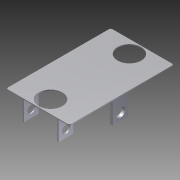
# Autodesk Inventor part: S114-electric
Saved by Autodesk Inventor 2011 SP1 (Build 150282100, 282)
## iProperties
Created: 2013-12-24
Part Number: S114-electric
Catalog Web Link: www.cadenas.de
Description: S Low Series electric-Low Capacity Standard Size Toggles -electric
Vendor: NKKSWITCHES
Document SubType Name: Modeling
Designer: PARTuser1
Manufacturer: NKKSWITCHES
Density: 1 g/cm^3
Category: PARTsolutions
Company: NKKSWITCHES
Title: S114-electric
Author: Cadenas PARTsolutions
Comments: Low Capacity Standard Size Toggles -electric
PSOL_IDENT_0: {$CADENAS_DATA\23d-libs\nkkswitches\toggle\s\parts\s_low_electric.prj},183 {VTYP=3D},{NB=S114-electr
PSOL_IDENT_1: ic},{LINA=S114-electric},{NN=S Low Series electric},{DATE=05.04.2013 12:38:11},{GEOMDATE=05.04.2013
PSOL_IDENT_2: 14:38:00},{VERSION=},{LINEID=10},{LINESUBID=-1},{WBVAR=}  {NB=S114-electric},{LINA=S114-electric},{K
PSOL_IDENT_3: T=DUMMY},{PN=S114},{MDL=S114}
CNS_NN: S Low Series electric
CNS_NT: Low Capacity Standard Size Toggles -electric
CNS_NB: S114-electric
CNS_NBSYN: $PN.-electric
CNS_LINA: S114-electric
CNS_PN: S114
CNS_MDL: S114
SUPPLIER: NKKSWITCHES
ARTICLENO: S114-electric
BOMINFO: S114-electric
CREATOR: CADENAS GmbH
Autodesk Inventor part; units mm, degrees
sketch "Sketch_1" plane through (0, 0, 0) normal (0, 1, 0) x (-1, 0, 0)
  line L0 (8.128, -12.954) -> (8.128, 12.954)
  arc A0 (8.128, 12.954) -> (7.62, 13.462) centre (7.62, 12.954) ccw
  line L1 (7.62, 13.462) -> (-7.62, 13.462)
  arc A1 (-7.62, 13.462) -> (-8.128, 12.954) centre (-7.62, 12.954) ccw
  line L2 (-8.128, 12.954) -> (-8.128, -12.954)
  arc A2 (-8.128, -12.954) -> (-7.62, -13.462) centre (-7.62, -12.954) ccw
  line L3 (-7.62, -13.462) -> (7.62, -13.462)
  arc A3 (7.62, -13.462) -> (8.128, -12.954) centre (7.62, -12.954) ccw
  circle A4 centre (0, 10.16) radius 3.048
  circle A5 centre (0, -10.16) radius 3.048
  constraints: 8 end point, 8 point on circle, 6 centre point
extrude "Extrusion1" add sketch "Sketch_1" along normal blind 0.254
sketch "Sketch_2" plane through (0, 0, 0) normal (0, 1, 0) x (1, 0, 0)
  line L0 (-4.6228, -12.7) -> (-4.318, -12.7)
  line L1 (-4.318, -12.7) -> (-4.318, -8.89)
  line L2 (-4.318, -8.89) -> (-4.6228, -8.89)
  line L3 (-4.6228, -8.89) -> (-4.6228, -12.7)
  constraints: 8 end point
extrude "Extrusion2" add sketch "Sketch_2" against normal blind 5.7658
sketch "Sketch_3" plane through (0, 0, 0) normal (0, 1, 0) x (1, 0, 0)
  line L0 (4.318, -12.7) -> (4.6228, -12.7)
  line L1 (4.6228, -12.7) -> (4.6228, -8.89)
  line L2 (4.6228, -8.89) -> (4.318, -8.89)
  line L3 (4.318, -8.89) -> (4.318, -12.7)
  constraints: 8 end point
extrude "Extrusion3" add sketch "Sketch_3" against normal blind 5.7658
sketch "Sketch4" plane through (-4.318, -5.7658, 8.89) normal (1, 0, 0) x (0, 0, -1)
  point P0 (-1.905, 1.9558)
hole "Drilling 1" at (-4.318, -3.81, 10.795) direction (-1, 0, 0) diameter 2.0066 depth 0.3048
sketch "Sketch5" plane through (4.318, -5.7658, 12.7) normal (-1, 0, 0) x (0, 0, 1)
  point P0 (-1.905, 1.9558)
hole "Drilling 2" at (4.318, -3.81, 10.795) direction (1, 0, 0) diameter 2.0066 depth 0.3048
sketch "Sketch_12" plane through (0, 0, 10.795) normal (0, 0, 1) x (1, 0, 0)
  line L0 (-4.6228, -1.27) -> (-4.9276, -1.27)
  arc A0 (-4.6228, -0.508) -> (-4.9276, -1.27) centre (-4.043, -1.1819) ccw
  line L1 (-4.6228, -0.508) -> (-4.6228, -1.27)
  line L2 (-4.6228, -1.27) -> (-4.9276, -1.27)
  constraints: 6 end point, 2 point on circle, 1 centre point
revolve "Revolution1" add sketch "Sketch_12" angle 360 about axis through (-4.6228, -1.27, 10.795) along (1, 0, 0)
sketch "Sketch_13" plane through (0, 0, 10.795) normal (0, 0, 1) x (1, 0, 0)
  line L0 (4.9276, -1.27) -> (4.6228, -1.27)
  line L1 (4.6228, -1.27) -> (4.6228, -0.508)
  arc A0 (4.9276, -1.27) -> (4.6228, -0.508) centre (4.043, -1.1819) ccw
  line L2 (4.9276, -1.27) -> (4.6228, -1.27)
  constraints: 6 end point, 2 point on circle, 1 centre point
revolve "Revolution2" add sketch "Sketch_13" angle 360 about axis through (4.9276, -1.27, 10.795) along (1, 0, 0)
sketch "Sketch_14" plane through (0, 0, 0) normal (0, 1, 0) x (-1, 0, 0)
  line L0 (7.8994, 1.9939) -> (7.112, 1.9939)
  line L1 (7.112, 1.9939) -> (7.112, -1.9939)
  line L2 (7.112, -1.9939) -> (7.8994, -1.9939)
  line L3 (7.8994, -1.9939) -> (7.8994, 1.9939)
  constraints: 8 end point
extrude "Extrusion4" add sketch "Sketch_14" against normal blind 5.7658
sketch "Sketch_15" plane through (0, 0, 0) normal (0, 1, 0) x (-1, 0, 0)
  line L0 (-7.112, 1.9939) -> (-7.8994, 1.9939)
  line L1 (-7.8994, 1.9939) -> (-7.8994, -1.9939)
  line L2 (-7.8994, -1.9939) -> (-7.112, -1.9939)
  line L3 (-7.112, -1.9939) -> (-7.112, 1.9939)
  constraints: 8 end point
extrude "Extrusion5" add sketch "Sketch_15" against normal blind 5.7658
sketch "Sketch10" plane through (-7.112, -5.7658, -1.9939) normal (1, 0, 0) x (0, 0, -1)
  point P0 (-1.9939, 1.9558)
hole "Drilling 3" at (-7.112, -3.81, 0) direction (-1, 0, 0) diameter 2.286 depth 0.7874
sketch "Sketch11" plane through (7.112, -5.7658, 1.9939) normal (-1, 0, 0) x (0, 0, 1)
  point P0 (-1.9939, 1.9558)
hole "Drilling 4" at (7.112, -3.81, 0) direction (1, 0, 0) diameter 2.286 depth 0.7874
ref_plane "to_body_XY" through (0, 0, 0) normal (0, -1, 0) x (1, 0, 0)
ref_plane "to_body_YZ" through (0, 0, 0) normal (1, 0, 0) x (0, 0, 1)
ref_plane "to_body_ZX" through (0, 0, 0) normal (0, 0, 1) x (0, -1, 0)
body "Solid1"
